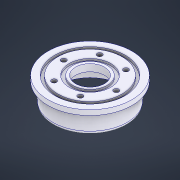
# Autodesk Inventor part: 020
Saved by Autodesk Inventor 2022 (Build 260153000, 153)
## iProperties
Created: 2021-11-03
Part Number: 020
Material: Polyethylene, High Density
Document SubType Name: Modeling
Designer: vinicius.miguel
Density: 0.952 g/cm^3
Appearance: Cool White
Author: vinicius.miguel
Autodesk Inventor part; units mm, degrees
ref_plane "YZ Plane" through (0, 0, 0) normal (1, 0, 0) x (0, 1, 0)
ref_plane "XZ Plane" through (0, 0, 0) normal (0, 1, 0) x (-1, 0, 0)
ref_plane "XY Plane" through (0, 0, 0) normal (0, 0, 1) x (1, 0, 0)
sketch "Sketch1" plane through (0, 0, 0) normal (0, 0, 1) x (1, 0, 0)
  line L0 (-36.75, 20) -> (-36.75, 3.182)
  arc A0 (-36.75, 3.182) -> (-31.318, 0.932) centre (-33.568, 3.182) ccw
  line L1 (-31.318, 0.932) -> (-14.25, 18)
  line L2 (-41.5, 25) -> (-41.5, 20)
  line L3 (-41.5, 20) -> (-36.75, 20)
  line L4 (0, 0) -> (0, 25) construction
  line L5 (0, 0) -> (-46.1303, 0) construction
  line L6 (-14.25, 18) -> (-14.25, 25)
  line L7 (-14.25, 25) -> (-41.5, 25)
  line L8 (-17, 25) -> (-17, 23)
  line L9 (-17, 23) -> (-20.5, 23)
  line L10 (-20.5, 23) -> (-20.5, 25)
  line L11 (-34.75, 25) -> (-34.75, 22.5)
  line L12 (-34.75, 22.5) -> (-31.75, 22.5)
  line L13 (-31.75, 22.5) -> (-31.75, 25)
  dimension "d0" = 28.5
  dimension "d2" = 18
  dimension "d4" = 83
  dimension "d5" = 73.5
  dimension "d20" = 25
  dimension "d21" = 135
  dimension "d22" = 5
  dimension "d23" = 34
  dimension "d24" = 3.5
  dimension "d25" = 2
  dimension "d37" = 3
  dimension "d38" = 2
  dimension "d39" = 2.5
  constraints: 28 end point, 6 perpendicular, 4 point on line, 4 vertical, 3 tangent, 2 point on circle, 1 centre point, 1 horizontal, 1 horizontal alignment
  measures "d0" diameter of L1.end L4
  measures "d2" vertical distance of L1.end L4.start
  measures "d4" diameter of L2 L4
  measures "d5" diameter of L0 L4
  measures "d20" distance from line of L7 L4.start
  measures "d21" angle of L1 L6
  measures "d22" distance of L2.start L2.end
  measures "d23" diameter of L8 L4
  measures "d24" distance of L8.end L9.end
  measures "d25" distance of L9.end L10.end
  measures "d37" distance of L11.end L12.end
  measures "d38" distance between parallel lines of L11 L0
  measures "d39" distance of L12.end L13.end
revolve "Revolution1" add sketch "Sketch1" angle 360 about axis through (0, 0, 0) along (0, 1, 0) contours L3 L2 L7 L11 L12 L13 L10 L9 L8 L6 L1 A0 L0
sketch "Sketch2" plane through (0, 25, 0) normal (0, 1, 0) x (1, 0, 0)
  point P0 (0, 0)
  point P1 (26, 0)
  dimension "d26" = 26
  constraints: 1 horizontal alignment
  measures "d26" distance of point (0, 0) point (26, 0)
hole "Hole1" at (26, 25, 0) direction (0, -1, 0) diameter 5 depth 6 tip angle 118
pattern_circular "Circular Pattern1" count 6 over 360 about axis through (0, 21.5, 0) along (0, 1, 0) of "Hole1"
body "Solid1"
